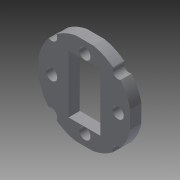
# Autodesk Inventor part: WG18FLANGECutDown
Saved by Autodesk Inventor 2014 (Build 180170000, 170)
## iProperties
Created: 2014-03-25
Part Number: WG18FLANGECutDown
Material: Generic
Document SubType Name: Modeling
Designer: jad211
Density: 1 g/cm^3
Appearance: Default
Author: jad211
Autodesk Inventor part; units mm, degrees
ref_plane "YZ Plane" through (0, 0, 0) normal (1, 0, 0) x (0, 1, 0)
ref_plane "XZ Plane" through (0, 0, 0) normal (0, 1, 0) x (-1, 0, 0)
ref_plane "XY Plane" through (0, 0, 0) normal (0, 0, 1) x (1, 0, 0)
sketch "Sketch3" plane through (0, 0, 0) normal (0, 0, 1) x (1, 0, 0)
  line L0 (-15.9263, -16.7) -> (16.0737, -16.7)
  line L1 (16.7744, -15.9999) -> (16.6729, 15.9999)
  line L2 (15.9735, 16.7) -> (-16.0265, 16.7)
  line L3 (-16.7272, 15.9999) -> (-16.6257, -15.9999)
  line L4 (-16.0265, 16.7) -> (-16.7272, 15.9999)
  line L5 (15.9735, 16.7) -> (16.6729, 15.9999)
  line L6 (16.7744, -15.9999) -> (16.0737, -16.7)
  line L7 (-16.6257, -15.9999) -> (-15.9263, -16.7)
  line L8 (-5.7625, -10.525) -> (5.7625, -10.525)
  line L9 (5.7625, -10.525) -> (5.7625, 10.525)
  line L10 (5.7625, 10.525) -> (-5.7625, 10.525)
  line L11 (-5.7625, 10.525) -> (-5.7625, -10.525)
  circle A0 centre (-12.159, 13.525) radius 2.045
  circle A1 centre (12.121, 13.525) radius 2.045
  circle A2 centre (-12.0777, -13.525) radius 2.045
  circle A3 centre (12.2023, -13.525) radius 2.045
  circle A4 centre (0, 0) radius 18.4 construction
  circle A5 centre (-12.1163, 0) radius 2.045
  circle A6 centre (0, 13.525) radius 2.045
  circle A7 centre (12.1637, 0) radius 2.045
  circle A8 centre (0, -13.525) radius 2.045
  dimension "d10" = 11.525
  dimension "d11" = 21.05
  dimension "d12" = 4.09
  dimension "d13" = 4.09
  dimension "d17" = 4.09
  dimension "d19" = 24.28
  dimension "d21" = 4.09
  dimension "d26" = 36.8
  dimension "d27" = 4.09
  dimension "d28" = 4.09
  dimension "d29" = 4.09
  dimension "d33" = 4.09
  dimension "d38" = 10.525
  dimension "d39" = 5.7625
  dimension "d45" = 33.4
  dimension "d46" = 33.4
  dimension "d47" = 32
  dimension "d48" = 32
  dimension "d49" = 32
  dimension "d50" = 32
  dimension "d52" = 3
  dimension "d53" = 3
  dimension "d55" = 3
  dimension "d56" = 3
  dimension "d57" = 3
  dimension "d59" = 3
  dimension "d60" = 5.7625
  dimension "d61" = 5.7625
  dimension "d62" = 6.3585
  dimension "d63" = 24.28
  dimension "d64" = 24.28
  dimension "d66" = 10.525
  dimension "d67" = 16.7
  constraints: 24 end point, 9 centre point, 6 parallel, 2 horizontal, 1 perpendicular
  measures "d10" distance of L10.end L9.end
  measures "d11" distance of L9.end L8.end
  measures "d12" diameter of A0
  measures "d13" diameter of A1
  measures "d17" diameter of A2
  measures "d19" distance of A1.centre A0.centre
  measures "d21" diameter of A3
  measures "d26" diameter of A4
  measures "d27" diameter of A5
  measures "d28" diameter of A6
  measures "d29" diameter of A7
  measures "d33" diameter of A8
  measures "d38" distance from line of point (0, 0) L8
  measures "d39" distance from line of point (0, 0) L9
  measures "d45" distance between parallel lines of L0 L2
  measures "d46" distance between parallel lines of L1 L3
  measures "d47" distance of L2.start L2.end
  measures "d48" distance of L3.start L3.end
  measures "d49" distance of L0.start L0.end
  measures "d50" distance of L1.start L1.end
  measures "d52" distance from line of A6.centre L10
  measures "d53" distance from line of A0.centre L10
  measures "d55" distance from line of L8 A8.centre
  measures "d56" distance from line of L8 A2.centre
  measures "d57" distance from line of L8 A3.centre
  measures "d59" distance from line of L10 A1.centre
  measures "d60" distance from line of A6.centre L9
  measures "d61" distance from line of L9 A8.centre
  measures "d62" distance from line of L9 A1.centre
  measures "d63" distance of A3.centre A2.centre
  measures "d64" distance of A5.centre A7.centre
  measures "d66" distance from line of L10 A5.centre
  measures "d67" distance from line of point (0, 0) L2
sketch "Sketch4" plane through (0, 0, 0) normal (0, 0, 1) x (1, 0, 0)
  circle A0 centre (0, 0) radius 17
  dimension "d32" = 34
  constraints: 1 centre point, 1 coincident
  measures "d32" diameter of A0
extrude "Extrusion3" add sketch "Sketch3" along normal blind 4.1
extrude "Extrusion4" cut sketch "Sketch4" along normal blind 4.1 keep common part
body "Solid3"
